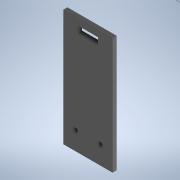
# Autodesk Inventor part: SP40V1 Chapa Base
Saved by Autodesk Inventor 2021.2 (Build 252289000, 289)
## iProperties
Created: 2026-08-24
Part Number: SP40V1 Chapa Base
Material: Generic
Document SubType Name: Sheet Metal
Designer: nelso
Density: 1 g/cm^3
Sheet Metal Rule: Default_mm
Appearance: Gray
Author: nelso
Autodesk Inventor part; units mm, degrees
ref_plane "YZ Plane" through (0, 0, 0) normal (1, 0, 0) x (0, 1, 0)
ref_plane "XZ Plane" through (0, 0, 0) normal (0, 1, 0) x (-1, 0, 0)
ref_plane "XY Plane" through (0, 0, 0) normal (0, 0, 1) x (1, 0, 0)
sketch "Sketch1" plane through (0, 0, 0) normal (0, 1, 0) x (-1, 0, 0)
  line L0 (20, 47.5) -> (-20, 47.5)
  line L1 (-20, 47.5) -> (-20, -47.5)
  line L2 (-20, -47.5) -> (20, -47.5)
  line L3 (20, -47.5) -> (20, 47.5)
  line L4 (20, 47.5) -> (-20, -47.5) construction
  line L5 (-20, 47.5) -> (20, -47.5) construction
  point P0 (0, 0)
  dimension "d0" = 40
  dimension "d1" = 95
  measures "d0" distance of L2.end L1.end
  measures "d1" distance of L1.end L0.end
extrude "Plate1" add sketch "Sketch1" along normal blind 3.2
sketch "Sketch2" plane through (0, 3.2, 0) normal (0, 1, 0) x (1, 0, 0)
  line L0 (-20, -47.5) -> (20, -47.5) projected
  line L1 (0, -47.5) -> (0, 32.5)
  line L2 (0, 32.5) -> (-10, 32.5)
  point P0 (0, 0)
  point P1 (10, 32.5)
  point P2 (10, 32.5)
  dimension "d3" = 80
  dimension "d4" = 10
  constraints: 4 end point, 2 coincident, 2 symmetric about line, 1 horizontal, 1 midpoint, 1 vertical
  measures "d3" distance of L1.start L1.end
  measures "d4" distance of L1.end L2.end
hole "Hole1" at (-10, 3.2, -32.5) at (10, 3.2, -32.5) direction (0, -1, 0) diameter 3.4 depth 3.2 tip angle 118 clearance for "Countersunk Flat Head Screw ISO 2009/7046" size "M3" standard "ISO"
sketch "Sketch4" plane through (0, 0, 0) normal (0, -1, 0) x (1, 0, 0)
  line L0 (-7.5, 39.559) -> (7.5, 39.559) projected
  line L1 (-7.5, 37.559) -> (-7.5, 39.559) projected
  line L2 (-7.5, 37.559) -> (7.5, 37.559) projected
  line L3 (7.5, 37.559) -> (7.5, 39.559) projected
  line L4 (8, 42.059) -> (-8, 42.059)
  line L5 (-8, 42.059) -> (-8, 37.059)
  line L6 (-8, 37.059) -> (8, 37.059)
  line L7 (8, 37.059) -> (8, 42.059)
  line L8 (8, 42.059) -> (-8, 37.059) construction
  line L9 (-8, 42.059) -> (8, 37.059) construction
  point P0 (0, 0)
  point P1 (0, 39.559)
  dimension "d12" = 16
  dimension "d13" = 5
  constraints: 12 end point, 3 midpoint, 2 parallel, 1 horizontal, 1 perpendicular
  measures "d12" distance of L6.end L5.end
  measures "d13" distance of L5.end L4.end
extrude "Cut1" cut sketch "Sketch4" against normal blind 3.2 contours L0 L3 L2 L1 | L7 L6 L5 L4
fillet "Corner Round1" radius 6 4 edges at (20, 1.6, 47.5) (-20, 1.6, 47.5) (20, 1.6, -47.5) (-20, 1.6, -47.5)
equation "\"d10\" = Thickness"
equation "\"d14\" = Thickness"
equation "\"d2\" = Thickness"
equation "\"BendReliefWidth\" = Thickness"
equation "\"BendReliefDepth\" = 0.5 * Thickness"
equation "\"CornerReliefSize\" = 4 * Thickness"
equation "\"MinimumRemnant\" = 2 * Thickness"
equation "\"TransitionRadius\" = BendRadius"
equation "\"JacobiRadiusSize\" = BendRadius"
equation "\"GapSize\" = Thickness"
equation "\"Thickness\" = 3.2"
equation "\"BendRadius\" = 1.516"
body "Solid1"
